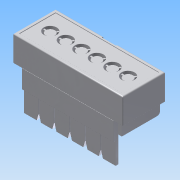
# Autodesk Inventor part: D2MG заглушка
Saved by Autodesk Inventor 2015 SP1 (Build 190203100, 203)
## iProperties
Created: 2017-11-05
Part Number: D2MG заглушка
Material: Типовые
Document SubType Name: Modeling
Designer: Влад
Density: 1 g/cm^3
Appearance: Белый пластик
Author: Влад
Autodesk Inventor part; units mm, degrees
ref_plane "YZ Plane" through (0, 0, 0) normal (1, 0, 0) x (0, 1, 0)
ref_plane "XZ Plane" through (0, 0, 0) normal (0, 1, 0) x (-1, 0, 0)
sketch "Эскиз1" plane through (0, 0, 0) normal (0, 0, 1) x (1, 0, 0)
  line L0 (-17.9, 6.95) -> (17.9, 6.95)
  line L1 (17.9, 6.95) -> (17.9, -6.95)
  line L2 (17.9, -6.95) -> (-17.9, -6.95)
  line L3 (-17.9, -6.95) -> (-17.9, 6.95)
  line L4 (-17.9, 6.95) -> (17.9, -6.95) construction
  line L5 (17.9, 6.95) -> (-17.9, -6.95) construction
  point P0 (0, 0)
  point P1 (0, 0)
  dimension "d0" = 35.8
  dimension "d1" = 13.9
  constraints: 12 end point, 2 parallel, 1 coincident, 1 horizontal, 1 midpoint, 1 perpendicular
  measures "d0" distance of L1.end L2.end
  measures "d1" distance of L0.end L1.end
extrude "Выдавливание1" add sketch "Эскиз1" along normal blind 1.7
sketch "Эскиз2" plane through (0, 0, 1.7) normal (0, 0, 1) x (1, 0, 0)
  line L0 (17.9, 6.95) -> (-17.9, 6.95) projected
  line L1 (-17.9, 6.95) -> (-17.9, -6.95) projected
  line L2 (-17.9, -6.95) -> (17.9, -6.95) projected
  line L3 (17.9, -6.95) -> (17.9, 6.95) projected
  line L4 (-16.9, 5.95) -> (16.9, 5.95)
  line L5 (16.9, 5.95) -> (16.9, -5.95)
  line L6 (16.9, -5.95) -> (-16.9, -5.95)
  line L7 (-16.9, -5.95) -> (-16.9, 5.95)
  point P0 (0, 0)
  dimension "d4" = 1
  dimension "d5" = 1
  dimension "d6" = 1
  dimension "d7" = 1
  constraints: 8 end point, 2 parallel, 1 horizontal, 1 perpendicular
  measures "d4" distance between parallel lines of L3 L5
  measures "d5" distance between parallel lines of L1 L7
  measures "d6" distance between parallel lines of L0 L4
  measures "d7" distance between parallel lines of L2 L6
extrude "Выдавливание2" cut sketch "Эскиз2" against normal blind 0.2 contours L4 L5 L6 L7
sketch "Эскиз3" plane through (0, 0, 1.5) normal (0, 0, 1) x (1, 0, 0)
  circle A0 centre (-12.7, 0) radius 2.1
  line L0 (-17.9, 6.95) -> (-17.9, -6.95) projected
  line L1 (17.9, 6.95) -> (-17.9, 6.95) projected
  line L2 (-12.7, 0) -> (-7.0579, 0) construction
  line L3 (-12.7, 0) -> (-14.8, 0) construction
  line L4 (-14.7851, -0.25) -> (-14.179, -0.25)
  line L5 (-14.7851, 0.25) -> (-14.179, 0.25)
  line L6 (-12.7, 0) -> (-11.458, 2.1512) construction
  line L7 (-12.7, 0) -> (-11.4765, -2.1192) construction
  line L8 (-11.874, 1.9307) -> (-12.177, 1.4059)
  line L9 (-11.441, 1.6807) -> (-11.744, 1.1559)
  line L10 (-12.177, -1.4059) -> (-11.874, -1.9307)
  line L11 (-11.744, -1.1559) -> (-11.441, -1.6807)
  arc A1 (-12.177, 1.4059) -> (-14.179, 0.25) centre (-12.7, 0) ccw
  arc A2 (-14.179, -0.25) -> (-12.177, -1.4059) centre (-12.7, 0) ccw
  arc A3 (-11.744, -1.1559) -> (-11.744, 1.1559) centre (-12.7, 0) ccw
  circle A4 centre (-7.62, 0) radius 2.1
  line L12 (-7.62, 0) -> (-9.72, 0) construction
  line L13 (-9.7051, -0.25) -> (-9.099, -0.25)
  line L14 (-9.7051, 0.25) -> (-9.099, 0.25)
  line L15 (-7.62, 0) -> (-6.378, 2.1512) construction
  line L16 (-7.62, 0) -> (-6.3965, -2.1192) construction
  line L17 (-6.794, 1.9307) -> (-7.097, 1.4059)
  line L18 (-6.361, 1.6807) -> (-6.664, 1.1559)
  line L19 (-7.097, -1.4059) -> (-6.794, -1.9307)
  line L20 (-6.664, -1.1559) -> (-6.361, -1.6807)
  arc A5 (-7.097, 1.4059) -> (-9.099, 0.25) centre (-7.62, 0) ccw
  arc A6 (-9.099, -0.25) -> (-7.097, -1.4059) centre (-7.62, 0) ccw
  arc A7 (-6.664, -1.1559) -> (-6.664, 1.1559) centre (-7.62, 0) ccw
  circle A8 centre (-2.54, 0) radius 2.1
  line L21 (-2.54, 0) -> (-4.64, 0) construction
  line L22 (-4.6251, -0.25) -> (-4.019, -0.25)
  line L23 (-4.6251, 0.25) -> (-4.019, 0.25)
  line L24 (-2.54, 0) -> (-1.298, 2.1512) construction
  line L25 (-2.54, 0) -> (-1.3165, -2.1192) construction
  line L26 (-1.714, 1.9307) -> (-2.017, 1.4059)
  line L27 (-1.281, 1.6807) -> (-1.584, 1.1559)
  line L28 (-2.017, -1.4059) -> (-1.714, -1.9307)
  line L29 (-1.584, -1.1559) -> (-1.281, -1.6807)
  arc A9 (-2.017, 1.4059) -> (-4.019, 0.25) centre (-2.54, 0) ccw
  arc A10 (-4.019, -0.25) -> (-2.017, -1.4059) centre (-2.54, 0) ccw
  arc A11 (-1.584, -1.1559) -> (-1.584, 1.1559) centre (-2.54, 0) ccw
  circle A12 centre (2.54, 0) radius 2.1
  line L30 (2.54, 0) -> (0.44, 0) construction
  line L31 (0.4549, -0.25) -> (1.061, -0.25)
  line L32 (0.4549, 0.25) -> (1.061, 0.25)
  line L33 (2.54, 0) -> (3.782, 2.1512) construction
  line L34 (2.54, 0) -> (3.7635, -2.1192) construction
  line L35 (3.366, 1.9307) -> (3.063, 1.4059)
  line L36 (3.799, 1.6807) -> (3.496, 1.1559)
  line L37 (3.063, -1.4059) -> (3.366, -1.9307)
  line L38 (3.496, -1.1559) -> (3.799, -1.6807)
  arc A13 (3.063, 1.4059) -> (1.061, 0.25) centre (2.54, 0) ccw
  arc A14 (1.061, -0.25) -> (3.063, -1.4059) centre (2.54, 0) ccw
  arc A15 (3.496, -1.1559) -> (3.496, 1.1559) centre (2.54, 0) ccw
  circle A16 centre (7.62, 0) radius 2.1
  line L39 (7.62, 0) -> (5.52, 0) construction
  line L40 (5.5349, -0.25) -> (6.141, -0.25)
  line L41 (5.5349, 0.25) -> (6.141, 0.25)
  line L42 (7.62, 0) -> (8.862, 2.1512) construction
  line L43 (7.62, 0) -> (8.8435, -2.1192) construction
  line L44 (8.446, 1.9307) -> (8.143, 1.4059)
  line L45 (8.879, 1.6807) -> (8.576, 1.1559)
  line L46 (8.143, -1.4059) -> (8.446, -1.9307)
  line L47 (8.576, -1.1559) -> (8.879, -1.6807)
  arc A17 (8.143, 1.4059) -> (6.141, 0.25) centre (7.62, 0) ccw
  arc A18 (6.141, -0.25) -> (8.143, -1.4059) centre (7.62, 0) ccw
  arc A19 (8.576, -1.1559) -> (8.576, 1.1559) centre (7.62, 0) ccw
  circle A20 centre (12.7, 0) radius 2.1
  line L48 (12.7, 0) -> (10.6, 0) construction
  line L49 (10.6149, -0.25) -> (11.221, -0.25)
  line L50 (10.6149, 0.25) -> (11.221, 0.25)
  line L51 (12.7, 0) -> (13.942, 2.1512) construction
  line L52 (12.7, 0) -> (13.9235, -2.1192) construction
  line L53 (13.526, 1.9307) -> (13.223, 1.4059)
  line L54 (13.959, 1.6807) -> (13.656, 1.1559)
  line L55 (13.223, -1.4059) -> (13.526, -1.9307)
  line L56 (13.656, -1.1559) -> (13.959, -1.6807)
  arc A21 (13.223, 1.4059) -> (11.221, 0.25) centre (12.7, 0) ccw
  arc A22 (11.221, -0.25) -> (13.223, -1.4059) centre (12.7, 0) ccw
  arc A23 (13.656, -1.1559) -> (13.656, 1.1559) centre (12.7, 0) ccw
  dimension "d10" = 4.2
  dimension "d16" = 5.2
  dimension "d20" = 6.95
  dimension "d29" = 0.25
  dimension "d30" = 0.25
  dimension "d31" = 120
  dimension "d32" = 120
  dimension "d33" = 0.25
  dimension "d34" = 0.25
  dimension "d35" = 0.25
  dimension "d36" = 0.25
  dimension "d39" = 5.08
  constraints: 110 end point, 36 point on circle, 18 centre point, 10 horizontal, 6 coincident, 6 parallel, 199 other
  measures "d16" distance from line of L0 L2.start
  measures "d20" distance from line of L1 L2.start
  measures "d29" distance between parallel lines of L3 L5
  measures "d30" distance between parallel lines of L4 L3
  measures "d31" angle of L3 L6
  measures "d32" angle of L3 L7
  measures "d33" distance between parallel lines of L7 L10
  measures "d34" distance between parallel lines of L11 L7
  measures "d35" distance between parallel lines of L6 L8
  measures "d36" distance between parallel lines of L9 L6
  measures "d39" distance of L3.start L12.start
extrude "Выдавливание3" cut sketch "Эскиз3" against normal through all contours A0 L11 A3 L9 | L8 A1 L5 A0 | A0 L4 A2 L10 | A4 L20 A7 L18 | L17 A5 L14 A4 | A4 L13 A6 L19 | A8 L29 A11 L27 | L26 A9 L23 A8 | A8 L22 A10 L28 | A12 L38 A15 L36 | L35 A13 L32 A12 | A12 L31 A14 L37 | A16 L47 A19 L45 | L44 A17 L41 A16 | A16 L40 A18 L46 | A20 L56 A23 L54 | L53 A21 L50 A20 | A20 L49 A22 L55
sketch "Эскиз4" plane through (0, 0, 1.5) normal (0, 0, 1) x (1, 0, 0)
  circle A0 centre (-12.7, 0) radius 2.1
  line L0 (-12.7, 0) -> (-9.12, 0) construction
  circle A1 centre (-7.62, 0) radius 2.1
  circle A2 centre (-2.54, 0) radius 2.1
  circle A3 centre (2.54, 0) radius 2.1
  circle A4 centre (7.62, 0) radius 2.1
  circle A5 centre (12.7, 0) radius 2.1
  point P0 (0, 0)
  dimension "d48" = 5.08
  constraints: 6 centre point, 2 end point, 2 horizontal, 1 coincident, 10 other
  measures "d48" distance of L0.start A1.centre
extrude "Выдавливание4" cut sketch "Эскиз4" against normal blind 0.5
sketch "Эскиз5" plane through (0, 0, 0) normal (0, 0, -1) x (-1, 0, 0)
  line L0 (-15, 5.45) -> (15, 5.45)
  line L1 (15, 5.45) -> (15, -5.45)
  line L2 (15, -5.45) -> (-15, -5.45)
  line L3 (-15, -5.45) -> (-15, 5.45)
  line L4 (17.9, -6.95) -> (17.9, 6.95) projected
  line L5 (-17.9, 6.95) -> (-17.9, -6.95) projected
  line L6 (17.9, 6.95) -> (-17.9, 6.95) projected
  line L7 (-17.9, -6.95) -> (17.9, -6.95) projected
  point P0 (0, 0)
  dimension "d55" = 2.9
  dimension "d56" = 2.9
  dimension "d57" = 1.5
  dimension "d58" = 1.5
  constraints: 8 end point, 2 parallel, 1 horizontal, 1 perpendicular
  measures "d55" distance between parallel lines of L4 L1
  measures "d56" distance between parallel lines of L5 L3
  measures "d57" distance between parallel lines of L0 L6
  measures "d58" distance between parallel lines of L7 L2
extrude "Выдавливание5" add sketch "Эскиз5" along normal blind 6.6
sketch "Эскиз6" plane through (0, 0, -6.6) normal (0, 0, -1) x (-1, 0, 0)
  line L0 (15, 6.95) -> (16.2, 6.95)
  line L1 (16.2, 6.95) -> (16.2, -5.55)
  line L2 (16.2, -5.55) -> (15, -5.55)
  line L3 (15, -5.55) -> (15, 6.95)
  line L4 (-16.2, 6.95) -> (-15, 6.95)
  line L5 (-15, 6.95) -> (-15, -5.55)
  line L6 (-15, -5.55) -> (-16.2, -5.55)
  line L7 (-16.2, -5.55) -> (-16.2, 6.95)
  line L8 (-17.9, 6.95) -> (-17.9, -6.95) projected
  line L9 (17.9, -6.95) -> (17.9, 6.95) projected
  line L10 (17.9, 6.95) -> (-17.9, 6.95) projected
  point P0 (0, 0)
  point P1 (15.6, 6.95)
  dimension "d61" = 1.2
  dimension "d62" = 12.5
  dimension "d63" = 1.2
  dimension "d64" = 12.5
  dimension "d65" = 2.9
  dimension "d66" = 2.9
  constraints: 16 end point, 4 parallel, 2 horizontal, 2 perpendicular, 2 point on line, 1 midpoint
  measures "d61" distance of L1.end L2.end
  measures "d62" distance of L0.end L1.end
  measures "d63" distance of L5.end L6.end
  measures "d64" distance of L4.end L5.end
  measures "d65" distance between parallel lines of L8 L5
  measures "d66" distance between parallel lines of L9 L3
extrude "Выдавливание6" add sketch "Эскиз6" along normal blind 4.5
sketch "Эскиз7" plane through (0, 0, -6.6) normal (0, 0, -1) x (-1, 0, 0)
  line L0 (15, -7.02) -> (-15, -7.02)
  line L1 (-15, -7.02) -> (-15, -5.45)
  line L2 (-15, -5.45) -> (15, -5.45)
  line L3 (15, -5.45) -> (15, -7.02)
  point P0 (0, 0)
  dimension "d69" = 1.57
  constraints: 8 end point, 2 parallel, 1 coincident, 1 horizontal, 1 perpendicular
  measures "d69" distance between parallel lines of L2 L0
extrude "Выдавливание7" add sketch "Эскиз7" along normal blind 6
sketch "Эскиз9" plane through (0, 0, -6.6) normal (0, 0, -1) x (-1, 0, 0)
  line L0 (-17.9, 6.95) -> (17.9, 6.95) projected
  line L1 (15, 5.45) -> (-15, 5.45)
  line L2 (-15, 5.45) -> (-15, 6.95)
  line L3 (-15, 6.95) -> (15, 6.95)
  line L4 (15, 6.95) -> (15, 5.45)
  point P0 (0, 0)
  constraints: 8 end point, 2 parallel, 1 horizontal, 1 perpendicular, 1 point on line
extrude "Выдавливание8" add sketch "Эскиз9" along normal blind 3.8
sketch "Эскиз10" plane through (-17.9, 6.95, 1.7) normal (0, 1, 0) x (1, 0, 0)
  line L0 (2.9, 1.7) -> (2.9, 12.1) projected
  line L1 (2.9, 1.7) -> (2.9, 12.1)
  line L2 (4.7, 12.1) -> (3.9, 1.7)
  line L3 (3.9, 1.7) -> (2.9, 1.7)
  line L4 (4.7, 12.1) -> (2.9, 12.1)
  line L5 (32.9, 12.1) -> (32.9, 1.7)
  line L6 (31.9, 1.7) -> (31.1, 12.1)
  line L7 (31.1, 12.1) -> (32.9, 12.1)
  line L8 (32.9, 12.1) -> (2.9, 12.1) projected
  line L9 (31.9, 1.7) -> (32.9, 1.7)
  line L10 (32.1, 1.7) -> (31.556, 1.7) projected
  point P0 (17.9, 1.7)
  dimension "d74" = 1.8
  dimension "d75" = 1
  dimension "d76" = 1.8
  dimension "d77" = 1
  constraints: 16 end point, 3 collinear, 1 vertical
  measures "d74" distance of L2.start L0.end
  measures "d75" distance of L2.end L0.start
  measures "d76" distance of L6.end L5.start
  measures "d77" distance of L6.start L5.end
extrude "Выдавливание9" cut sketch "Эскиз10" against normal blind 1.6
sketch "Эскиз11" plane through (0, 0, 1.7) normal (0, 0, 1) x (1, 0, 0)
  line L0 (-2.35, 6.95) -> (2.35, 6.95)
  line L1 (2.35, 6.95) -> (2.35, 6.45)
  line L2 (2.35, 6.45) -> (-2.35, 6.45)
  line L3 (-2.35, 6.45) -> (-2.35, 6.95)
  line L4 (-17.9, 6.95) -> (-17.9, -6.95) projected
  line L5 (17.9, -6.95) -> (17.9, 6.95) projected
  line L6 (17.9, 6.95) -> (-17.9, 6.95) projected
  point P0 (0, 0)
  point P1 (0, 6.95)
  dimension "d80" = 4.7
  dimension "d81" = 0.5
  dimension "d82" = 15.55
  constraints: 8 end point, 2 midpoint, 2 parallel, 1 horizontal, 1 perpendicular
  measures "d80" distance of L1.end L2.end
  measures "d81" distance of L0.end L1.end
  measures "d82" distance between parallel lines of L4 L3
extrude "Выдавливание10" cut sketch "Эскиз11" against normal blind 6.6
ref_plane "РабПлоскость1" through (-1.5, -6.95, 1.7) normal (-1, 0, 0) x (0, 0, 1)
sketch "Эскиз12" plane through (-1.5, -6.95, 1.7) normal (-1, 0, 0) x (0, 0, 1)
  line L0 (-6.6, 13.9) -> (-6.6, 14.5)
  line L1 (-6.6, 14.5) -> (-8.6, 13.9)
  line L2 (-8.6, 13.9) -> (-6.6, 13.9)
  point P0 (-1.7, 6.95)
  dimension "d88" = 0.6
  dimension "d89" = 2
  constraints: 6 end point, 1 vertical
  measures "d88" distance of L0.start L0.end
  measures "d89" distance of L1.end L0.start
extrude "Выдавливание11" add sketch "Эскиз12" against normal blind 3
sketch "Эскиз13" plane through (0, 0, -12.6) normal (0, 0, -1) x (-1, 0, 0)
  line L0 (15, -6.35) -> (10.3, -6.35)
  line L1 (10.3, -6.35) -> (10.3, -5.45)
  line L2 (10.3, -5.45) -> (15, -5.45)
  line L3 (15, -5.45) -> (15, -6.35)
  line L4 (-15, -5.45) -> (15, -5.45) projected
  line L5 (4.88, -6.35) -> (0.18, -6.35)
  line L6 (0.18, -6.35) -> (0.18, -5.45)
  line L7 (0.18, -5.45) -> (4.88, -5.45)
  line L8 (4.88, -5.45) -> (4.88, -6.35)
  line L9 (9.94, -6.35) -> (5.24, -6.35)
  line L10 (5.24, -6.35) -> (5.24, -5.45)
  line L11 (5.24, -5.45) -> (9.94, -5.45)
  line L12 (9.94, -5.45) -> (9.94, -6.35)
  line L13 (-0.18, -6.35) -> (-4.88, -6.35)
  line L14 (-4.88, -6.35) -> (-4.88, -5.45)
  line L15 (-4.88, -5.45) -> (-0.18, -5.45)
  line L16 (-0.18, -5.45) -> (-0.18, -6.35)
  line L17 (-5.24, -6.35) -> (-9.94, -6.35)
  line L18 (-9.94, -6.35) -> (-9.94, -5.45)
  line L19 (-9.94, -5.45) -> (-5.24, -5.45)
  line L20 (-5.24, -5.45) -> (-5.24, -6.35)
  line L21 (-10.3, -6.35) -> (-15, -6.35)
  line L22 (-15, -6.35) -> (-15, -5.45)
  line L23 (-15, -5.45) -> (-10.3, -5.45)
  line L24 (-10.3, -5.45) -> (-10.3, -6.35)
  point P0 (0, 0)
  point P1 (12.65, -5.45)
  dimension "d92" = 4.7
  dimension "d93" = 0.9
  dimension "d94" = 4.7
  dimension "d95" = 0.9
  dimension "d96" = 4.7
  dimension "d97" = 0.9
  dimension "d98" = 4.7
  dimension "d99" = 0.9
  dimension "d100" = 4.7
  dimension "d101" = 0.9
  dimension "d102" = 0.36
  dimension "d103" = 0.36
  dimension "d104" = 0.36
  dimension "d105" = 0.36
  dimension "d106" = 4.7
  dimension "d107" = 0.9
  dimension "d108" = 0.36
  constraints: 48 end point, 12 parallel, 6 horizontal, 6 perpendicular, 3 point on line, 1 midpoint
  measures "d92" distance of L1.end L2.end
  measures "d93" distance of L0.end L1.end
  measures "d94" distance of L6.end L7.end
  measures "d95" distance of L5.end L6.end
  measures "d96" distance of L10.end L11.end
  measures "d97" distance of L9.end L10.end
  measures "d98" distance of L14.end L15.end
  measures "d99" distance of L13.end L14.end
  measures "d100" distance of L18.end L19.end
  measures "d101" distance of L17.end L18.end
  measures "d102" distance between parallel lines of L12 L1
  measures "d103" distance between parallel lines of L8 L10
  measures "d104" distance between parallel lines of L16 L6
  measures "d105" distance between parallel lines of L14 L20
  measures "d106" distance of L22.end L23.end
  measures "d107" distance of L21.end L22.end
  measures "d108" distance between parallel lines of L24 L18
extrude "Выдавливание12" add sketch "Эскиз13" along normal blind 7
sketch "Эскиз14" plane through (0.18, -6.35, -12.6) normal (0, -1, 0) x (1, 0, 0)
  line L0 (10.62, -7) -> (10.12, -5.2)
  line L1 (10.62, -7) -> (10.12, -7)
  line L2 (10.12, -7) -> (10.12, -5.2)
  line L3 (10.2449, -7) -> (9.0207, -7) construction
  line L4 (9.76, -7) -> (5.06, -7) projected
  line L5 (5.56, -7) -> (5.06, -5.2)
  line L6 (5.56, -7) -> (5.06, -7)
  line L7 (5.06, -7) -> (5.06, -5.2)
  line L8 (0.5, -7) -> (0, -5.2)
  line L9 (0.5, -7) -> (0, -7)
  line L10 (0, -7) -> (0, -5.2)
  line L11 (-4.56, -7) -> (-5.06, -5.2)
  line L12 (-4.56, -7) -> (-5.06, -7)
  line L13 (-5.06, -7) -> (-5.06, -5.2)
  line L14 (-9.62, -7) -> (-10.12, -5.2)
  line L15 (-9.62, -7) -> (-10.12, -7)
  line L16 (-10.12, -7) -> (-10.12, -5.2)
  line L17 (-10.48, -7) -> (-10.48, -5.2)
  line L18 (-10.48, -5.2) -> (-10.98, -7)
  line L19 (-10.98, -7) -> (-10.48, -7)
  line L20 (-5.42, -7) -> (-5.42, -5.2)
  line L21 (-5.42, -5.2) -> (-5.92, -7)
  line L22 (-5.92, -7) -> (-5.42, -7)
  line L23 (-0.36, -7) -> (-0.36, -5.2)
  line L24 (-0.36, -5.2) -> (-0.86, -7)
  line L25 (-0.86, -7) -> (-0.36, -7)
  line L26 (4.7, -7) -> (4.7, -5.2)
  line L27 (4.7, -5.2) -> (4.2, -7)
  line L28 (4.2, -7) -> (4.7, -7)
  line L29 (9.76, -7) -> (9.76, -5.2)
  line L30 (9.76, -5.2) -> (9.26, -7)
  line L31 (9.26, -7) -> (9.76, -7)
  point P0 (-0.18, 12.6)
  point P1 (5.1849, -7)
  point P2 (0.1249, -7)
  point P3 (-4.9351, -7)
  point P4 (-9.9951, -7)
  dimension "d111" = 0.5
  dimension "d112" = 1.8
  dimension "d115" = 5.06
  dimension "d122" = 1.8
  dimension "d123" = 0.5
  dimension "d126" = 5.06
  constraints: 62 end point, 11 point on line, 3 horizontal, 1 coincident, 1 perpendicular, 1 vertical, 56 other
  measures "d111" distance of L0.start L1.end
  measures "d112" distance of L1.end L2.end
  measures "d115" distance of L0.start L5.start
  measures "d122" distance of L17.start L17.end
  measures "d123" distance of L18.end L17.start
  measures "d126" distance of L17.end L21.start
extrude "Выдавливание13" cut sketch "Эскиз14" against normal through all
fillet "Сопряжение1" radius 0.2 4 edges at (-17.9, -6.95, -2.45) (17.9, -6.95, -2.45) (17.9, 6.95, -2.45) (-17.9, 6.95, -2.45)
fillet "Сопряжение2" radius 0.35 9 edges at (17.8414, -6.8914, 1.7) (17.9, 0, 1.7) (17.8414, 6.8914, 1.7) (10.025, 6.95, 1.7) (-17.8414, -6.8914, 1.7) (-17.9, 0, 1.7) (-17.8414, 6.8914, 1.7) (-10.025, 6.95, 1.7) (0, -6.95, 1.7)
fillet "Сопряжение3" radius 1 2 edges at (-15.6, 6.95, -11.1) (15.6, 6.95, -11.1)
fillet "Сопряжение4" radius 0.05 72 edges at (0, 5.95, 1.7) (-16.9, 0, 1.7) (0, -5.95, 1.7) (16.9, 0, 1.7) (11.65, 1.8187, 1.5) (11.65, -1.8187, 1.5) (14.7851, 0.25, 1.5) (13.75, -1.8187, 1.5) (10.6, 0, 1.5) (6.57, -1.8187, 1.5) (9.7051, 0.25, 1.5) (6.57, 1.8187, 1.5) (8.67, -1.8187, 1.5) (5.52, 0, 1.5) (1.49, -1.8187, 1.5) (4.6251, 0.25, 1.5) (1.49, 1.8187, 1.5) (3.59, -1.8187, 1.5) (0.44, 0, 1.5) (-3.59, -1.8187, 1.5) (-0.4549, 0.25, 1.5) (-3.59, 1.8187, 1.5) (-1.49, -1.8187, 1.5) (-4.64, 0, 1.5) (-8.67, -1.8187, 1.5) (-5.5349, 0.25, 1.5) (-8.67, 1.8187, 1.5) (-6.57, -1.8187, 1.5) (-9.72, 0, 1.5) (-13.75, -1.8187, 1.5) (-10.6149, 0.25, 1.5) (-13.75, 1.8187, 1.5) (-14.8, 0, 1.5) (-11.65, -1.8187, 1.5) (0, 6.45, 1.7) (17.8414, -6.8914, -6.6) (16.35, -6.95, -6.6) (17.8414, 6.8914, -6.6) (16.95, 6.95, -6.6) (17.9, 0, -6.6) (15, -7.02, -9.6) (15, -6.685, -12.6) (15, -6.35, -16.1) (0, -7.02, -12.6) (10.55, -6.35, -18.7) (10.3, -6.35, -15.2) (9.94, -6.35, -15.2) (9.69, -6.35, -18.7) (5.49, -6.35, -18.7) (5.24, -6.35, -15.2) (4.88, -6.35, -15.2) (4.63, -6.35, -18.7) (0.43, -6.35, -18.7) (0.18, -6.35, -15.2) (-0.18, -6.35, -15.2) (-0.43, -6.35, -18.7) (-4.88, -6.35, -15.2) (-5.24, -6.35, -15.2) (-5.49, -6.35, -18.7) (-4.63, -6.35, -18.7) (-9.69, -6.35, -18.7) (-10.55, -6.35, -18.7) (-10.3, -6.35, -15.2) (-9.94, -6.35, -15.2) (-15, -6.35, -16.1) (-15, -6.685, -12.6) (-15, -7.02, -9.6) (-17.8414, -6.8914, -6.6) (-17.9, 0, -6.6) (-17.8414, 6.8914, -6.6) (-16.95, 6.95, -6.6) (-16.35, -6.95, -6.6)
